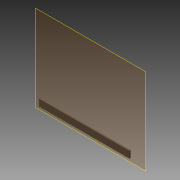
# Autodesk Inventor part: Hidder_Right
Saved by Autodesk Inventor 2014 SP1 (Build 180222100, 222)
## iProperties
Created: 2015-04-07
Part Number: Hidder_Right
Material: MDF Medium Density Fiberboard
Document SubType Name: Modeling
Designer: tuleu
Density: 0.8 g/cm^3
Appearance: Cardboard - Corrugated
Author: tuleu
Autodesk Inventor part; units mm, degrees
ref_plane "YZ Plane" through (0, 0, 0) normal (1, 0, 0) x (0, 1, 0)
ref_plane "XZ Plane" through (0, 0, 0) normal (0, 1, 0) x (-1, 0, 0)
ref_plane "Work Plane1" through (0, 0, 0) normal (0, 0, 1) x (1, 0, 0)
sketch "Sketch1" plane through (0, 0, 0) normal (0, 0, 1) x (1, 0, 0)
  line L0 (-2085, -287.5) -> (-607.5, -287.5) construction
  line L1 (-2085, -287.5) -> (-2085, 862.5) construction
  line L2 (-2085, -187.5) -> (-1905, -187.5) construction
  line L3 (-757.5, -187.5) -> (-757.5, -387.5) construction
  line L4 (-2085, -187.5) -> (-757.5, -187.5)
  line L5 (-757.5, -187.5) -> (-757.5, -287.5)
  line L6 (-757.5, -287.5) -> (-2085, -287.5)
  line L7 (-2085, -287.5) -> (-2085, -187.5)
  point P0 (0, 0)
  constraints: 8 end point, 2 parallel, 1 horizontal, 1 midpoint, 1 perpendicular
ref_plane "Work Plane2" through (-2100, -287.5, 19) normal (0, 0, 1) x (1, 0, 0)
extrude "Extrusion1" add sketch "Sketch1" along normal up to surface (19 mm away)
body "Solid1"
